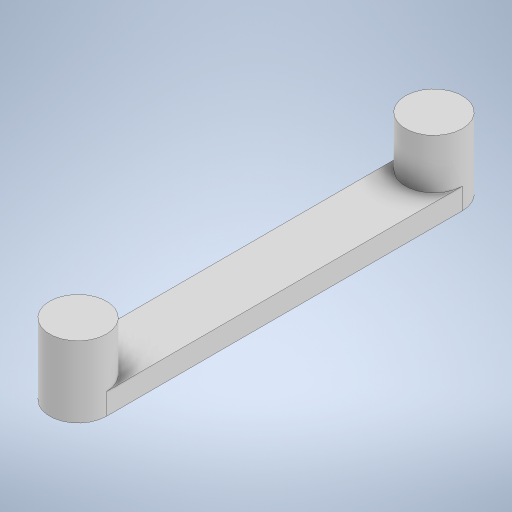
# Autodesk Inventor part: Base
Saved by Autodesk Inventor 2024.3 (Build 283343000, 343)
## iProperties
Created: 2024-11-06
Part Number: Base
Material: Generic
Document SubType Name: Modeling
Designer: wszaf
Density: 1 g/cm^3
Appearance: Default
Author: wszaf
Autodesk Inventor part; units mm, degrees
ref_plane "YZ Plane" through (0, 0, 0) normal (1, 0, 0) x (0, 1, 0)
ref_plane "XZ Plane" through (0, 0, 0) normal (0, 1, 0) x (-1, 0, 0)
ref_plane "XY Plane" through (0, 0, 0) normal (0, 0, 1) x (1, 0, 0)
sketch "Sketch1" plane through (0, 0, 0) normal (0, 1, 0) x (-1, 0, 0)
  circle A0 centre (4, -4) radius 4
  circle A1 centre (4, -54) radius 4
  line L0 (8, 0) -> (0, 0)
  line L1 (0, 0) -> (0, -58)
  line L2 (0, -58) -> (8, -58)
  line L3 (8, -58) -> (8, 0)
  point P0 (8, -54)
  point P1 (8, -4)
  point P2 (0, -4)
  point P3 (0, -54)
  dimension "d0" = 8
  dimension "d1" = 8
  dimension "d2" = 50
  constraints: 8 end point, 5 tangent, 2 centre point, 2 parallel, 1 coincident, 1 horizontal, 1 perpendicular
  measures "d0" diameter of A0
  measures "d1" diameter of A1
  measures "d2" distance of A0.centre A1.centre
extrude "Extrusion1" add sketch "Sketch1" along normal blind 7 contours A0 | A1
extrude "Extrusion2" add sketch "Sketch1" against normal blind 3 contours A0 | L3 A1 L1 A0 | A1
equation "\"d0\" = Internal_Diameter"
equation "\"d1\" = Internal_Diameter"
equation "\"d2\" = Center_Distance"
equation "\"d3\" = Pin_Height"
equation "\"Center_Distance\" = 50"
equation "\"Internal_Diameter\" = 8"
equation "\"Pin_Height\" = 7"
body "Solid1"
